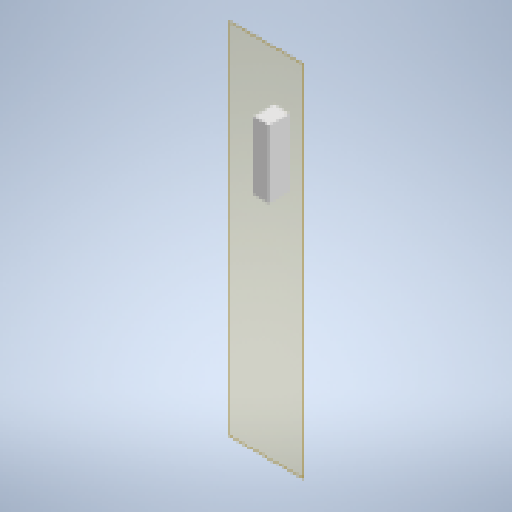
# Autodesk Inventor part: Avionics
Saved by Autodesk Inventor 2027.1 (Build 311270010, 270A)
## iProperties
Created: 2026-09-10
Part Number: Avionics
Material: Generic
Document SubType Name: Modeling
Designer: PWYNNE
Density: 1 g/cm^3
Appearance: Default
Author: PWYNNE
Autodesk Inventor part; units mm, degrees
ref_plane "YZ Plane" through (0, 0, 0) normal (1, 0, 0) x (0, 1, 0)
ref_plane "XZ Plane" through (0, 0, 0) normal (0, 1, 0) x (-1, 0, 0)
ref_plane "XY Plane" through (0, 0, 0) normal (0, 0, 1) x (1, 0, 0)
ref_plane "Work Plane1" through (0, 0, 0) normal (0, 0, 1) x (1, 0, 0)
sketch "Sketch1" plane through (0, 0, 0) normal (0, 0, 1) x (1, 0, 0)
  line L0 (-90, 404.1414) -> (-60, 404.1414) projected
  line L1 (-60, 404.1414) -> (-60, 434.1414) projected
  line L2 (-60, 434.1414) -> (-90, 434.1414) projected
  line L3 (-90, 434.1414) -> (-90, 404.1414) projected
  line L4 (-60, 734.2829) -> (-60, 762.2829)
  line L5 (-60, 284.1414) -> (-60, 374.1414) projected
  line L6 (-60, 374.1414) -> (-60, 404.1414) construction
  line L7 (-60, 284.1414) -> (-90, 284.1414) construction
  spline S0 degree 3 poles (-10, 350) (-10, 360.2589) (-10.8658, 370.3929) (-14.4668, 392.6865) (-17.5742, 404.4656) (-26.8496, 431.6444) (-33.7108, 445.9172) (-45.2886, 465.4296) (-50.0022, 472.1002) (-55.3711, 478.3258) (-56.2225, 479.2687) (-59.645, 482.8719) (-62.119, 485.0608) (-66.6024, 488.033) (-68.2627, 488.7862) (-70.2419, 489.4323) (-70.852, 489.5961) (-71.4777, 489.7181) knots 0.305224 0.305224 0.305224 0.305224 0.919495 0.919495 1.689795 1.689795 2.84097 2.84097 3.625871 3.625871 3.775317 3.775317 4.231595 4.231595 4.59332 4.59332 4.735389 4.735389 4.735389 4.735389 projected
  line L8 (-10, -490) -> (-10, 350) projected
  line L9 (-60, 284.1414) -> (-30, 284.1414)
  line L10 (-30, 284.1414) -> (-30, 414.1414)
  line L11 (-30, 414.1414) -> (-60, 414.1414)
  line L12 (-60, 414.1414) -> (-60, 284.1414)
  point P0 (0, 0)
  dimension "d0" = 30
  dimension "d1" = 130
  constraints: 10 end point, 2 parallel, 1 horizontal, 1 perpendicular, 1 vertical, 2 other
  measures "d0" distance of L11.end L10.end
  measures "d1" distance of L10.end L9.end
extrude "Extrusion1" add sketch "Sketch1" along normal blind 40 contours L1 L11 L10 L9 L5 L12
body "Solid1"
